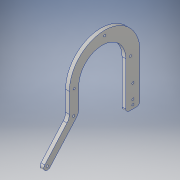
# Autodesk Inventor part: Hook Plate
Saved by Autodesk Inventor 2019.4 (Build 234330000, 330)
## iProperties
Created: 2020-03-10
Part Number: Hook Plate
Material: Aluminum 6061
Document SubType Name: Modeling
Designer: admin
Density: 2.7 g/cm^3
Appearance: Aluminum - Flat
Author: admin
Autodesk Inventor part; units mm, degrees
ref_plane "YZ Plane" through (0, 0, 0) normal (1, 0, 0) x (0, 1, 0)
ref_plane "XZ Plane" through (0, 0, 0) normal (0, 1, 0) x (-1, 0, 0)
ref_plane "XY Plane" through (0, 0, 0) normal (0, 0, 1) x (1, 0, 0)
sketch "Sketch1" plane through (0, 0, 0) normal (1, 0, 0) x (0, 1, 0)
  line L0 (0, 0) -> (100, 0)
  line L1 (0, 0) -> (0, 30)
  line L2 (0, 30) -> (100, 30)
  arc A0 (100, 30) -> (100, 130) centre (100, 80) ccw
  line L3 (100, 130) -> (50, 130)
  line L4 (50, 150) -> (100, 150)
  circle A1 centre (8, 15) radius 2.2
  circle A2 centre (18, 15) radius 2.2
  line L5 (8, 15) -> (48, 15) construction
  circle A3 centre (48, 15) radius 2.2
  circle A4 centre (50, 141) radius 2.2
  circle A5 centre (100, 140) radius 2.2
  circle A6 centre (165, 75) radius 2.2
  circle A7 centre (100, 20) radius 2.2
  line L6 (165, 75) -> (175, 75) construction
  line L7 (50, 130) -> (-25, 196.1438)
  line L8 (-25, 196.1438) -> (-15.0784, 207.3938)
  line L9 (-15.0784, 207.3938) -> (50, 150)
  line L10 (50, 150) -> (50, 141) construction
  circle A8 centre (-14.4142, 196.808) radius 2.2
  arc A9 (100, 0) -> (100, 150) centre (100, 75) ccw
  point P0 (0, 15)
  dimension "d0" = 30
  dimension "d1" = 100
  dimension "d2" = 100
  dimension "d3" = 50
  dimension "d4" = 50
  dimension "d5" = 4.4
  dimension "d6" = 4.4
  dimension "d9" = 10
  dimension "d10" = 40
  dimension "d11" = 4.4
  dimension "d12" = 8
  dimension "d13" = 50
  dimension "d14" = 4.4
  dimension "d16" = 11
  dimension "d17" = 4.4
  dimension "d18" = 4.4
  dimension "d19" = 4.4
  dimension "d20" = 10
  dimension "d22" = 10
  dimension "d23" = 10
  dimension "d24" = 100
  dimension "d27" = 15
  dimension "d28" = 100
  dimension "d29" = 4.4
  dimension "d30" = 7.5
  dimension "d31" = 7.5
  dimension "d32" = 50
  dimension "d34" = 20
  constraints: 22 end point, 10 centre point, 5 point on circle, 4 horizontal, 4 tangent, 2 perpendicular, 2 point on line, 2 vertical, 1 coincident, 1 line through centre, 1 midpoint, 1 parallel
  measures "d0" distance of L0.start L1.end
  measures "d1" distance of L1.end L2.end
  measures "d2" distance of L0.start L0.end
  measures "d3" distance of L4.start L4.end
  measures "d4" radius of A0
  measures "d5" diameter of A1
  measures "d6" diameter of A2
  measures "d9" distance of L5.start A2.centre
  measures "d10" distance of L5.start L5.end
  measures "d11" diameter of A3
  measures "d12" distance from line of L5.start L1
  measures "d13" distance of L3.start L3.end
  measures "d14" diameter of A4
  measures "d16" distance from line of L3 L10.end
  measures "d17" diameter of A5
  measures "d18" diameter of A6
  measures "d19" diameter of A7
  measures "d20" distance from line of L4 A5.centre
  measures "d22" distance of L6.end L6.start
  measures "d23" distance from line of L2 A7.centre
  measures "d24" distance from line of L1 A7.centre
  measures "d27" distance of L7.end L8.end
  measures "d28" distance of L3.end L7.end
  measures "d29" diameter of A8
  measures "d30" distance from line of L7 A8.centre
  measures "d31" distance from line of A8.centre L8
  measures "d32" distance from line of L10 A5.centre
  measures "d34" distance between parallel lines of L3 L4
extrude "Extrusion1" add sketch "Sketch1" along normal blind 8
fillet "Fillet1" radius 20 2 edges at (4, 50, 150) (4, 50, 130)
fillet "Fillet2" radius 7.5 2 edges at (4, -25, 196.1438) (4, -15.0784, 207.3938)
fillet "Fillet3" radius 7.5 2 edges at (4, 0, 30) (4, 0, 0)
equation "\"d24\" = d1"
equation "\"d32\" = d3"
body "Solid1"
